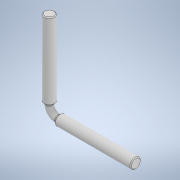
# Autodesk Inventor part: Część22
Saved by Autodesk Inventor 2021 (Build 250183000, 183)
## iProperties
Created: 2023-11-01
Part Number: Część22
Material: Ogólny
Document SubType Name: Modeling
Designer: Jakub
Density: 1 g/cm^3
Appearance: Domyślna
Author: Jakub
Autodesk Inventor part; units mm, degrees
ref_plane "YZ Plane" through (0, 0, 0) normal (1, 0, 0) x (0, 1, 0)
ref_plane "XZ Plane" through (0, 0, 0) normal (0, 1, 0) x (-1, 0, 0)
ref_plane "XY Plane" through (0, 0, 0) normal (0, 0, 1) x (1, 0, 0)
sketch "Szkic1" plane through (0, 0, 0) normal (0, 0, 1) x (1, 0, 0)
  line L0 (0, 0) -> (0, 5)
  line L1 (0, 5) -> (5, 5)
  line L2 (0, 0) -> (-4.2426, 4.2426)
  line L3 (0, 0) -> (6, 0) construction
  line L4 (-4.2426, 4.2426) -> (4.2426, -4.2426)
  line L5 (-4.2426, 4.2426) -> (9.8995, 18.3848)
  line L6 (4.2426, -4.2426) -> (18.3848, 9.8995)
  line L7 (-2, 6.4853) -> (0, 6.4853)
  line L8 (0, 6.4853) -> (2, 6.4853)
  line L9 (6.4853, -2) -> (6.4853, 0)
  line L10 (6.4853, 0) -> (6.4853, 2)
  line L11 (6.4853, 0) -> (5, 0)
  line L12 (0, 6.4853) -> (0, 5)
  arc A0 (0, 5) -> (5, 0) centre (5, 5) ccw
  line L13 (1.4645, 1.4645) -> (0.0503, 0.0503)
  line L14 (1.4645, 1.4645) -> (3.4645, 1.4645) construction
  arc A1 (-2, 5) -> (0.0503, 0.0503) centre (5, 5) ccw
  arc A2 (0.0503, 0.0503) -> (5, -2) centre (5, 5) ccw
  line L15 (1.4645, 1.4645) -> (2.8787, 2.8787)
  arc A3 (2, 5) -> (2.8787, 2.8787) centre (5, 5) ccw
  arc A4 (2.8787, 2.8787) -> (5, 2) centre (5, 5) ccw
  line L16 (5, 2) -> (6.4853, 2)
  line L17 (2, 5) -> (2, 6.4853)
  line L18 (-2, 5) -> (-2, 6.4853)
  line L19 (5, -2) -> (6.4853, -2)
  line L20 (-4.2426, 4.2426) -> (-26.5165, 26.5165)
  line L21 (4.2426, -4.2426) -> (26.5165, -26.5165)
  line L22 (26.5165, -26.5165) -> (61.8718, 8.8388)
  line L23 (-26.5165, 26.5165) -> (8.8388, 61.8718)
  line L24 (-3, 50.033) -> (0, 50.033)
  line L25 (0, 50.033) -> (3, 50.033)
  line L26 (50.033, -3) -> (50.033, 0)
  line L27 (50.033, 0) -> (50.033, 3)
  line L28 (50.033, 3) -> (6.4853, 3)
  line L29 (6.4853, 3) -> (6.4853, 2)
  line L30 (50.033, -3) -> (6.4853, -3)
  line L31 (6.4853, -3) -> (6.4853, -2)
  line L32 (-3, 50.033) -> (-3, 6.4853)
  line L33 (-3, 6.4853) -> (-2, 6.4853)
  line L34 (3, 50.033) -> (3, 6.4853)
  line L35 (3, 6.4853) -> (2, 6.4853)
  dimension "d0" = 5
  dimension "d1" = 5
  dimension "d2" = 6
  dimension "d3" = 135
  dimension "d4" = 12
  dimension "d5" = 20
  dimension "d6" = 20
  dimension "d7" = 2
  dimension "d8" = 2
  dimension "d10" = 2
  dimension "d11" = 135
  dimension "d12" = 2
  dimension "d13" = 31.5
  dimension "d14" = 31.5
  dimension "d15" = 50
  dimension "d16" = 50
  dimension "d17" = 3
  dimension "d18" = 3
  constraints: 72 end point, 15 point on line, 13 point on circle, 11 perpendicular, 6 horizontal, 5 centre point, 5 coincident, 3 vertical, 2 concentric, 2 equal length, 1 collinear, 1 parallel
  measures "d0" distance of L0.start L0.end
  measures "d1" distance of L0.end L1.end
  measures "d2" distance of L0.start L2.end
  measures "d3" angle of L3 L2
  measures "d4" distance of L2.end L4.end
  measures "d5" distance of L2.end L5.end
  measures "d6" distance of L4.end L6.end
  measures "d7" distance of L7.end L8.end
  measures "d8" distance of L9.end L10.end
  measures "d10" distance of L13.start L13.end
  measures "d11" angle of L13 L14
  measures "d12" distance of L13.start L15.end
  measures "d13" distance of L2.end L20.end
  measures "d14" distance of L4.end L21.end
  measures "d15" distance of L21.end L22.end
  measures "d16" distance of L20.end L23.end
  measures "d17" distance of L24.end L25.end
  measures "d18" distance of L26.end L27.end
sketch "Szkic2" plane through (0, 0, 0) normal (0, 0, 1) x (1, 0, 0)
  line L0 (0, 0) -> (0, 5)
  line L1 (0, 5) -> (5, 5)
  line L2 (0, 0) -> (-4.2426, 4.2426)
  line L3 (0, 0) -> (6, 0) construction
  line L4 (-4.2426, 4.2426) -> (4.2426, -4.2426)
  line L5 (-4.2426, 4.2426) -> (9.8995, 18.3848)
  line L6 (4.2426, -4.2426) -> (18.3848, 9.8995)
  line L7 (-2, 6.4853) -> (0, 6.4853)
  line L8 (0, 6.4853) -> (2, 6.4853)
  line L9 (6.4853, -2) -> (6.4853, 0)
  line L10 (6.4853, 0) -> (6.4853, 2)
  line L11 (6.4853, 0) -> (5, 0)
  line L12 (0, 6.4853) -> (0, 5)
  arc A0 (0, 5) -> (5, 0) centre (5, 5) ccw
  line L13 (1.4645, 1.4645) -> (0.0503, 0.0503)
  line L14 (1.4645, 1.4645) -> (3.4645, 1.4645) construction
  arc A1 (-2, 5) -> (0.0503, 0.0503) centre (5, 5) ccw
  arc A2 (0.0503, 0.0503) -> (5, -2) centre (5, 5) ccw
  line L15 (1.4645, 1.4645) -> (2.8787, 2.8787)
  arc A3 (2, 5) -> (2.8787, 2.8787) centre (5, 5) ccw
  arc A4 (2.8787, 2.8787) -> (5, 2) centre (5, 5) ccw
  line L16 (5, 2) -> (6.4853, 2)
  line L17 (2, 5) -> (2, 6.4853)
  line L18 (-2, 5) -> (-2, 6.4853)
  line L19 (5, -2) -> (6.4853, -2)
  line L20 (-4.2426, 4.2426) -> (-26.5165, 26.5165)
  line L21 (4.2426, -4.2426) -> (26.5165, -26.5165)
  line L22 (26.5165, -26.5165) -> (61.8718, 8.8388)
  line L23 (-26.5165, 26.5165) -> (8.8388, 61.8718)
  line L24 (-3, 50.033) -> (0, 50.033)
  line L25 (0, 50.033) -> (3, 50.033)
  line L26 (50.033, -3) -> (50.033, 0)
  line L27 (50.033, 0) -> (50.033, 3)
  line L28 (50.033, 3) -> (6.4853, 3)
  line L29 (6.4853, 3) -> (6.4853, 2)
  line L30 (50.033, -3) -> (6.4853, -3)
  line L31 (6.4853, -3) -> (6.4853, -2)
  line L32 (-3, 50.033) -> (-3, 6.4853)
  line L33 (-3, 6.4853) -> (-2, 6.4853)
  line L34 (3, 50.033) -> (3, 6.4853)
  line L35 (3, 6.4853) -> (2, 6.4853)
  dimension "d19" = 5
  dimension "d20" = 5
  dimension "d21" = 6
  dimension "d22" = 135
  dimension "d23" = 12
  dimension "d24" = 20
  dimension "d25" = 20
  dimension "d26" = 2
  dimension "d27" = 2
  dimension "d28" = 2
  dimension "d29" = 135
  dimension "d30" = 2
  dimension "d31" = 31.5
  dimension "d32" = 31.5
  dimension "d33" = 50
  dimension "d34" = 50
  dimension "d35" = 3
  dimension "d36" = 3
  constraints: 72 end point, 15 point on line, 13 point on circle, 11 perpendicular, 6 horizontal, 5 centre point, 5 coincident, 3 vertical, 2 concentric, 2 equal length, 1 collinear, 1 parallel
  measures "d19" distance of L0.start L0.end
  measures "d20" distance of L0.end L1.end
  measures "d21" distance of L0.start L2.end
  measures "d22" angle of L3 L2
  measures "d23" distance of L2.end L4.end
  measures "d24" distance of L2.end L5.end
  measures "d25" distance of L4.end L6.end
  measures "d26" distance of L7.end L8.end
  measures "d27" distance of L9.end L10.end
  measures "d28" distance of L13.start L13.end
  measures "d29" angle of L13 L14
  measures "d30" distance of L13.start L15.end
  measures "d31" distance of L2.end L20.end
  measures "d32" distance of L4.end L21.end
  measures "d33" distance of L21.end L22.end
  measures "d34" distance of L20.end L23.end
  measures "d35" distance of L24.end L25.end
  measures "d36" distance of L26.end L27.end
extrude "Wyciągnięcie proste1" add sketch "Szkic1" along normal mid plane 4 contours A1 L18 L7 L12 L0 | L0 A0 L13 A1 | L12 L8 L17 L1 | L1 A3 L15 A0 | L13 A0 L11 L9 L19 A2 | L15 A4 L16 L10 L11 A0
sketch "Szkic3" plane through (0, 0, 2) normal (0, 0, 1) x (1, 0, 0)
  line L0 (0, 0) -> (0, 5)
  line L1 (0, 5) -> (5, 5)
  line L2 (0, 0) -> (-4.2426, 4.2426)
  line L3 (0, 0) -> (6, 0) construction
  line L4 (-4.2426, 4.2426) -> (4.2426, -4.2426)
  line L5 (-4.2426, 4.2426) -> (9.8995, 18.3848)
  line L6 (4.2426, -4.2426) -> (18.3848, 9.8995)
  line L7 (-2, 6.4853) -> (0, 6.4853)
  line L8 (0, 6.4853) -> (2, 6.4853)
  line L9 (6.4853, -2) -> (6.4853, 0)
  line L10 (6.4853, 0) -> (6.4853, 2)
  line L11 (6.4853, 0) -> (5, 0)
  line L12 (0, 6.4853) -> (0, 5)
  arc A0 (0, 5) -> (5, 0) centre (5, 5) ccw
  line L13 (1.4645, 1.4645) -> (0.0503, 0.0503)
  line L14 (1.4645, 1.4645) -> (3.4645, 1.4645) construction
  arc A1 (-2, 5) -> (0.0503, 0.0503) centre (5, 5) ccw
  arc A2 (0.0503, 0.0503) -> (5, -2) centre (5, 5) ccw
  line L15 (1.4645, 1.4645) -> (2.8787, 2.8787)
  arc A3 (2, 5) -> (2.8787, 2.8787) centre (5, 5) ccw
  arc A4 (2.8787, 2.8787) -> (5, 2) centre (5, 5) ccw
  line L16 (5, 2) -> (6.4853, 2)
  line L17 (2, 5) -> (2, 6.4853)
  line L18 (-2, 5) -> (-2, 6.4853)
  line L19 (5, -2) -> (6.4853, -2)
  line L20 (-4.2426, 4.2426) -> (-26.5165, 26.5165)
  line L21 (4.2426, -4.2426) -> (26.5165, -26.5165)
  line L22 (26.5165, -26.5165) -> (61.8718, 8.8388)
  line L23 (-26.5165, 26.5165) -> (8.8388, 61.8718)
  line L24 (-3, 50.033) -> (0, 50.033)
  line L25 (0, 50.033) -> (3, 50.033)
  line L26 (50.033, -3) -> (50.033, 0)
  line L27 (50.033, 0) -> (50.033, 3)
  line L28 (50.033, 3) -> (6.4853, 3)
  line L29 (6.4853, 3) -> (6.4853, 2)
  line L30 (50.033, -3) -> (6.4853, -3)
  line L31 (6.4853, -3) -> (6.4853, -2)
  line L32 (-3, 50.033) -> (-3, 6.4853)
  line L33 (-3, 6.4853) -> (-2, 6.4853)
  line L34 (3, 50.033) -> (3, 6.4853)
  line L35 (3, 6.4853) -> (2, 6.4853)
  dimension "d39" = 5
  dimension "d40" = 5
  dimension "d41" = 6
  dimension "d42" = 135
  dimension "d43" = 12
  dimension "d44" = 20
  dimension "d45" = 20
  dimension "d46" = 2
  dimension "d47" = 2
  dimension "d48" = 2
  dimension "d49" = 135
  dimension "d50" = 2
  dimension "d51" = 31.5
  dimension "d52" = 31.5
  dimension "d53" = 50
  dimension "d54" = 50
  dimension "d55" = 3
  dimension "d56" = 3
  constraints: 72 end point, 15 point on line, 13 point on circle, 11 perpendicular, 6 horizontal, 5 centre point, 5 coincident, 3 vertical, 2 concentric, 2 equal length, 1 collinear, 1 parallel
  measures "d39" distance of L0.start L0.end
  measures "d40" distance of L0.end L1.end
  measures "d41" distance of L0.start L2.end
  measures "d42" angle of L3 L2
  measures "d43" distance of L2.end L4.end
  measures "d44" distance of L2.end L5.end
  measures "d45" distance of L4.end L6.end
  measures "d46" distance of L7.end L8.end
  measures "d47" distance of L9.end L10.end
  measures "d48" distance of L13.start L13.end
  measures "d49" angle of L13 L14
  measures "d50" distance of L13.start L15.end
  measures "d51" distance of L2.end L20.end
  measures "d52" distance of L4.end L21.end
  measures "d53" distance of L21.end L22.end
  measures "d54" distance of L20.end L23.end
  measures "d55" distance of L24.end L25.end
  measures "d56" distance of L26.end L27.end
extrude "Wyciągnięcie proste2" add sketch "Szkic3" along normal blind 1 and the other way blind 5 contours L33 L32 L24 L25 L34 L5 | L5 L34 L35 L8 L7 | L9 L10 L29 L28 L6 | L6 L28 L27 L26 L30 L31
fillet "Zaokrąglenie1" radius 3 8 edges at (3, 28.2591, 3) (-3, 28.2591, 3) (3, 28.2591, -3) (-3, 28.2591, -3) (28.2591, 3, -3) (28.2591, -3, 3) (28.2591, 3, 3) (28.2591, -3, -3)
fillet "Zaokrąglenie2" radius 2 16 edges at (3.8519, 2.2284, -2) (2.2284, 3.8519, -2) (5.7426, 2, -2) (2, 5.7426, -2) (-2, 5.7426, -2) (5.7426, -2, -2) (-1.4672, 2.3212, -2) (2.3212, -1.4672, -2) (5.7426, -2, 2) (-2, 5.7426, 2) (-1.4672, 2.3212, 2) (2.3212, -1.4672, 2) (2, 5.7426, 2) (5.7426, 2, 2) (3.8519, 2.2284, 2) (2.2284, 3.8519, 2)
fillet "Zaokrąglenie3" radius 1 19 edges at (2, 6.4853, 0) (1.4142, 6.4853, -1.4142) (1.4142, 6.4853, 1.4142) (0, 6.4853, -2) (0, 6.4853, 2) (-1.4142, 6.4853, -1.4142) (-1.4142, 6.4853, 1.4142) (-2, 6.4853, -0.0001) (-2, 6.4853, 0.0001) (6.4853, 0, -2) (6.4853, 0, 2) (6.4853, 1.4142, -1.4142) (6.4853, -1.4142, -1.4142) (6.4853, -1.4142, 1.4142) (6.4853, 1.4142, 1.4142) (6.4853, -2, 0.0001) (6.4853, 2, 0.0001) (6.4853, -2, -0.0001) (6.4853, 2, -0.0001)
chamfer "Faza1" distance 0.5 angle 45 16 edges at (3, 50.033, 0) (2.1213, 50.033, 2.1213) (2.1213, 50.033, -2.1213) (0, 50.033, 3) (0, 50.033, -3) (-2.1213, 50.033, 2.1213) (-2.1213, 50.033, -2.1213) (-3, 50.033, 0) (50.033, 3, 0) (50.033, 2.1213, 2.1213) (50.033, 2.1213, -2.1213) (50.033, 0, 3) (50.033, 0, -3) (50.033, -2.1213, 2.1213) (50.033, -2.1213, -2.1213) (50.033, -3, 0)
